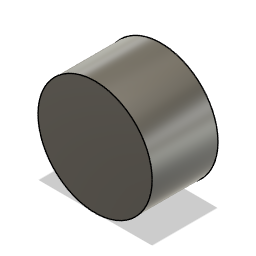
tapas_tubos v3 (Autodesk Fusion 360 design; units mm, degrees)
Autodesk Fusion 360 part; units mm, degrees
sketch "Boceto1" plane through (0, 0, 0) normal (0, 1, 0) x (1, 0, 0)
  circle A0 centre (0, 0) radius 7.25
  circle A1 centre (0, 0) radius 10.25
  circle A2 centre (0, 0) radius 13.25
  dimension "d1" = 14.5
  dimension "d2" = 20.5
  dimension "d17" = 3
  constraint coincident A0.centre A1.centre
  constraint concentric A0 A1
  measures "d1" diameter of A0
  measures "d2" diameter of A1
  measures "d17" distance of A1 A2
sketch "Boceto2" plane through (0, 0, 0) normal (0, 1, 0) x (1, 0, 0)
  circle A0 centre (0, 0) radius 10.25
  circle A1 centre (0, 0) radius 2
  dimension "d7" = 20.5
  dimension "d8" = 4
  constraint coincident A0.centre A1.centre
  measures "d7" diameter of A0
  measures "d8" diameter of A1
sketch "Boceto3" plane through (0, 0, 0) normal (0, 0, 1) x (1, 0, 0)
  spline S0 degree 5 poles (-2, 25) (-2.1979, 23.8996) (-2.5982, 21.7436) (-3.2127, 18.6435) (-4.0601, 14.7825) (-5.1702, 10.4479) (-6.3378, 6.668) (-7.5715, 3.5272) (-8.8809, 1.1182) (-10.2748, -0.4741) (-11.7577, -1.2066) (-13.0133, -1.123) (-13.9924, -0.6995) (-14.6614, -0.2594) (-15, 0) knots 0 0 0 0 0 0 0.1 0.2 0.3 0.4 0.5 0.6 0.7 0.8 0.9 1 1 1 1 1 1
  spline S1 degree 5 poles (2, 25) (2.1979, 23.8996) (2.5982, 21.7436) (3.2127, 18.6435) (4.0601, 14.7825) (5.1702, 10.4479) (6.3378, 6.668) (7.5715, 3.5272) (8.8809, 1.1182) (10.2748, -0.4741) (11.7577, -1.2066) (13.0133, -1.123) (13.9924, -0.6995) (14.6614, -0.2594) (15, 0) knots 0 0 0 0 0 0 0.1 0.2 0.3 0.4 0.5 0.6 0.7 0.8 0.9 1 1 1 1 1 1
  point P0 (-10, 0)
  point P1 (10, 0)
sketch "Boceto4" plane through (0, 0, 0) normal (0, 0, 1) x (1, 0, 0)
  circle A0 centre (0, 0) radius 10
  circle A1 centre (0, 0) radius 13
  dimension "d18" = 20
  dimension "d19" = 3
  constraint coincident A0.centre A1.centre
  measures "d18" diameter of A0
  measures "d19" distance of A0 A1
extrude "Extruir7" add sketch "Boceto4" along normal blind 10 makes body 1
ref_plane "PlanoDeObra1" through (0, 0, 5) normal (0, 0, 1) x (1, 0, 0)
sketch "Boceto5" plane through (0, 0, 5) normal (0, 0, 1) x (1, 0, 0)
  circle A0 centre (0, 0) radius 10
  circle A1 centre (0, 0) radius 11.5
  dimension "d23" = 20
  dimension "d24" = 23
  constraint coincident A0.centre A1.centre
  measures "d23" diameter of A0
  measures "d24" diameter of A1
extrude "Extruir8" cut sketch "Boceto5" along normal mid plane 2 bodies 1
extrude "Extruir9" add 1 faces at (11.9144, -1.1427, 10) along direction (0, 0, 1) blind 5 on bodies 1 bodies 1
ref_plane "PlanoDeObra2" through (0, 0, 40) normal (0, 0, 1) x (1, 0, 0)
sketch "Boceto6" plane through (0, 0, 40) normal (0, 0, 1) x (1, 0, 0)
  circle A0 centre (0, 0) radius 2
  dimension "d30" = 4
  constraint coincident A0.centre origin
  measures "d30" diameter of A0
sketch "Boceto7" plane through (0, 0, 15) normal (0, 0, 1) x (1, 0, 0)
  circle A0 centre (0, 0) radius 10
  circle A1 centre (0, 0) radius 13
  circle A2 centre (0, 0) radius 13
  constraint coincident A0.centre A1.centre
loft "Solevación2" add profiles "Boceto6", "Boceto7" section 1 section 2 bodies 1
extrude "Extruir10" cut sketch "Boceto6" against normal blind 71 bodies 1
ref_plane "PlanoDeObra3" through (0, 0, 10) normal (0, 0, -1) x (-1, 0, 0)
split "Dividir1" by plane through (0, 0, 10) normal (0, 0, -1) bodies 1 makes body 2 at (12.9354, -1.2944, 3.3333)
move_face "CarasDesfase1" offset -0.3 2 faces at (9.9503, -0.9957, 1.3333) (9.9503, 0.9957, 8.6667) on bodies 2
ref_plane "PlanoDeObra4" through (0, 0, 4) normal (0, 0, -1) x (-1, 0, 0)
split "Dividir2" by plane through (0, 0, 4) normal (0, 0, -1) bodies 2 makes body 3 at (12.9354, 1.2944, 2.6667)
extrude "Extruir11" add 2 faces at (12.4516, 0.6458, 4) (11.0188, 1.083, 4) along direction (0, 0, 1) blind 6 on bodies 3 bodies 3
combine "Combinar1" operation add target body 1 tool bodies 3
extrude "Extruir12" cut 1 faces at (9.861, 2.5062, 10) along direction (0, 0, -1) blind 8 from surface at -5 on bodies 1 bodies 1
extrude "Extruir13" cut sketch "Boceto5" along normal mid plane 3 bodies 1
copy_body "CopiarPegarCuerpos1" bodies 1 makes body 4
move_body "Desplazar1" bodies 4 to x (1, 0, 0) y (0, 1, 0) z (0, 0, 1) at (34, 0, 0)
split "Dividir3" by plane through (0, 0, 10) normal (0, 0, -1) bodies 4 makes body 5 at (46.9838, 0.648, 3.3333)
delete_body "QuitarCuerpo1" bodies 4
delete_body "QuitarCuerpo2" bodies 2
sketch "Boceto8" plane through (0, 0, 10) normal (0, 0, 1) x (1, 0, 0)
  circle A0 centre (34, 0) radius 13
  circle A1 centre (34, 0) radius 10.3
  line L0 (34, -13) -> (34, 13) construction
  line L1 (47, 0) -> (21, 0) construction
  circle A2 centre (34, 0) radius 13
  constraint coincident A0 L0.start
  constraint coincident A0 L0.end
  constraint vertical L0
  constraint coincident A0 L1.start
  constraint coincident A0 L1.end
  constraint perpendicular L0 L1
  constraint concentric A0 A2
  constraint coincident L0.start A2
extrude "Extruir14" add sketch "Boceto8" along normal blind 5 contours A0 A2 | A1 bodies 5
extrude "Extruir6" [suppressed]
hidden bodies 1
named bodies: "taponfinal", "prueba (1)", "prueba (1) (1)", "taporecto"
